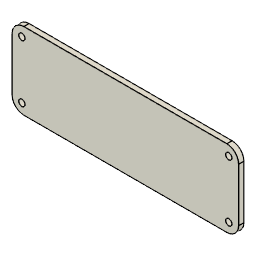
Head Door (Autodesk Fusion 360 design; units mm, degrees)
part number: 2026-07-07-16-47-09-751
Autodesk Fusion 360 part; units mm, degrees
sketch "Sketch1" plane through (0, 0, 0) normal (0, 0, 1) x (1, 0, 0)
  line L0 (0, 0) -> (115, 0)
  line L1 (115, 0) -> (115, 39)
  line L2 (115, 39) -> (0, 39)
  line L3 (0, 39) -> (0, 0)
  circle A0 centre (5, 34) radius 1.6
  circle A1 centre (5, 5) radius 1.6
  circle A2 centre (110, 5) radius 1.6
  circle A3 centre (110, 34) radius 1.6
  dimension "d1" = 115
  dimension "d2" = 39
  dimension "d3" = 3.2
  dimension "d4" = 5
  dimension "d5" = 5
  dimension "d6" = 3.2
  dimension "d7" = 5
  dimension "d8" = 5
  dimension "d9" = 3.2
  dimension "d10" = 3.2
  dimension "d11" = 5
  dimension "d12" = 5
  dimension "d13" = 5
  dimension "d14" = 5
  constraint horizontal L0
  constraint vertical L1
  constraint horizontal L2
  constraint vertical L3
  constraint coincident L0.start L3.end
  measures "d1" distance of L0.start L0.end
  measures "d2" distance of L0.start L2.end
  measures "d3" diameter of A0
  measures "d4" distance of L3 A0.centre
  measures "d5" distance of L2 A0.centre
  measures "d6" diameter of A1
  measures "d7" distance of L0 A1.centre
  measures "d8" distance of L3 A1.centre
  measures "d9" diameter of A2
  measures "d10" diameter of A3
  measures "d11" distance of L0 A2.centre
  measures "d12" distance of L1 A2.centre
  measures "d13" distance of L1 A3.centre
  measures "d14" distance of L2 A3.centre
extrude "Extrude1" add sketch "Sketch1" along normal blind 2.7
fillet "Fillet1" radius 6 4 edges at (115, 39, 1.35) (115, 0, 1.35) (0, 39, 1.35) (0, 0, 1.35)
